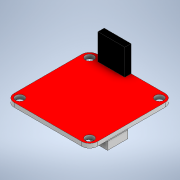
# Autodesk Inventor part: razor_sketch
Saved by Autodesk Inventor 2020 (Build 240168000, 168)
## iProperties
Created: 2024-03-26
Part Number: razor_sketch
Material: Типовые
Document SubType Name: Modeling
Designer: 4s
Density: 1 g/cm^3
Appearance: По умолчанию
Author: 4s
Autodesk Inventor part; units mm, degrees
ref_plane "YZ Plane" through (0, 0, 0) normal (1, 0, 0) x (0, 1, 0)
ref_plane "XZ Plane" through (0, 0, 0) normal (0, 1, 0) x (-1, 0, 0)
ref_plane "XY Plane" through (0, 0, 0) normal (0, 0, 1) x (1, 0, 0)
sketch "Эскиз1" plane through (0, 0, 0) normal (0, 1, 0) x (-1, 0, 0)
  line L0 (13, 16) -> (-13, 16)
  line L1 (-16, 13) -> (-16, -13)
  line L2 (-13, -16) -> (13, -16)
  line L3 (16, -13) -> (16, 13)
  line L4 (0, 0) -> (32.4367, 0) construction
  line L5 (0, 0) -> (0, -34.7046) construction
  circle A0 centre (13.4, -13.4) radius 1.625
  circle A1 centre (-13.4, -13.4) radius 1.625
  circle A2 centre (13.4, 13.4) radius 1.625
  circle A3 centre (-13.4, 13.4) radius 1.625
  arc A4 (16, 13) -> (13, 16) centre (13, 13) ccw
  arc A5 (13, -16) -> (16, -13) centre (13, -13) ccw
  arc A6 (-16, -13) -> (-13, -16) centre (-13, -13) ccw
  arc A7 (-13, 16) -> (-16, 13) centre (-13, 13) ccw
  point P0 (-16, -16)
  point P1 (-16, 16)
  point P2 (16, -16)
  dimension "d0" = 32
  dimension "d1" = 32
  dimension "d2" = 3.25
  dimension "d3" = 26.8
  dimension "d4" = 26.8
  dimension "d5" = 3
  constraints: 12 end point, 8 centre point, 8 point on circle, 8 tangent, 6 point on line, 3 equal radius, 3 symmetric about line, 2 horizontal, 2 parallel, 1 perpendicular, 1 vertical, 5 other
  measures "d0" distance of point (16, -16) point (-16, -16)
  measures "d1" distance of point (-16, -16) point (-16, 16)
  measures "d2" diameter of A0
  measures "d3" distance of A1.centre A0.centre
  measures "d4" distance of A2.centre A0.centre
  measures "d5" radius of A4
extrude "Выдавливание1" add sketch "Эскиз1" along normal blind 1.6
sketch "Эскиз2" plane through (0, 1.6, 0) normal (0, 1, 0) x (1, 0, 0)
  line L0 (-10.4, 13.6) -> (-0.1, 13.6)
  line L1 (-0.1, 13.6) -> (-0.1, 16)
  line L2 (-0.1, 16) -> (-10.4, 16)
  line L3 (-10.4, 16) -> (-10.4, 13.6)
  line L4 (-13, -16) -> (13, -16) construction
  arc A0 (13, -16) -> (16, -13) centre (13, -13) ccw construction
  line L5 (16, -13) -> (16, 13) construction
  arc A1 (16, 13) -> (13, 16) centre (13, 13) ccw construction
  line L6 (13, 16) -> (-13, 16) construction
  arc A2 (-13, 16) -> (-16, 13) centre (-13, 13) ccw construction
  line L7 (-16, 13) -> (-16, -13) construction
  arc A3 (-16, -13) -> (-13, -16) centre (-13, -13) ccw construction
  circle A4 centre (13.4, 13.4) radius 1.625 construction
  circle A5 centre (13.4, -13.4) radius 1.625 construction
  circle A6 centre (-13.4, -13.4) radius 1.625 construction
  circle A7 centre (-13.4, 13.4) radius 1.625 construction
  point P0 (0, 0)
  dimension "d8" = 10.3
  dimension "d9" = 2.4
  dimension "d10" = 5.6
  constraints: 8 end point, 2 parallel, 1 collinear, 1 horizontal, 1 perpendicular
  measures "d8" distance of L2.end L1.end
  measures "d9" distance of L1.end L0.end
  measures "d10" distance between parallel lines of L3 L7
extrude "Выдавливание2" add sketch "Эскиз2" along normal blind 10
sketch "Эскиз3" plane through (0, 0, 0) normal (0, -1, 0) x (1, 0, 0)
  line L0 (16.3, 9.4) -> (9.3, 9.4)
  line L1 (9.3, 9.4) -> (9.3, 1.6)
  line L2 (9.3, 1.6) -> (16.3, 1.6)
  line L3 (16.3, 1.6) -> (16.3, 9.4)
  line L4 (-13, 16) -> (13, 16) construction
  arc A0 (-13, 16) -> (-16, 13) centre (-13, 13) ccw construction
  line L5 (-16, -13) -> (-16, 13) construction
  arc A1 (-16, -13) -> (-13, -16) centre (-13, -13) ccw construction
  line L6 (13, -16) -> (-13, -16) construction
  arc A2 (13, -16) -> (16, -13) centre (13, -13) ccw construction
  line L7 (16, 13) -> (16, -13) construction
  arc A3 (16, 13) -> (13, 16) centre (13, 13) ccw construction
  circle A4 centre (13.4, -13.4) radius 1.625 construction
  circle A5 centre (13.4, 13.4) radius 1.625 construction
  circle A6 centre (-13.4, 13.4) radius 1.625 construction
  circle A7 centre (-13.4, -13.4) radius 1.625 construction
  point P0 (0, 0)
  dimension "d13" = 0.3
  dimension "d14" = 7.8
  dimension "d15" = 7
  dimension "d16" = 6.6
  constraints: 8 end point, 2 parallel, 1 horizontal, 1 perpendicular
  measures "d13" distance between parallel lines of L3 L7
  measures "d14" distance between parallel lines of L2 L0
  measures "d15" distance between parallel lines of L1 L3
  measures "d16" distance between parallel lines of L4 L0
extrude "Выдавливание3" add sketch "Эскиз3" along normal blind 3
